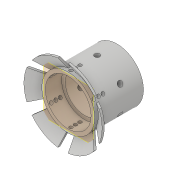
# Autodesk Inventor part: 01_Autofocus_Magnet_holder_v0
Saved by Autodesk Inventor 2019.4 (Build 234330000, 330)
## iProperties
Created: 2020-10-26
Part Number: 01_Autofocus_Magnet_holder_v0
Material: Generic
Document SubType Name: Modeling
Designer: diederichbenedict
Density: 1 g/cm^3
Appearance: Default
Author: diederichbenedict
Autodesk Inventor part; units mm, degrees
ref_plane "YZ Plane" through (0, 0, 0) normal (1, 0, 0) x (0, 1, 0)
ref_plane "XZ Plane" through (0, 0, 0) normal (0, 1, 0) x (-1, 0, 0)
ref_plane "XY Plane" through (0, 0, 0) normal (0, 0, 1) x (1, 0, 0)
ref_plane "Work Plane1" through (0, 0, 0) normal (0, 0, 1) x (1, 0, 0)
sketch "Sketch1" plane through (0, 0, 0) normal (0, 0, 1) x (1, 0, 0)
  circle A0 centre (0, 0) radius 12.5 construction
  circle A1 centre (0, 0) radius 12.65
  circle A2 centre (0, 0) radius 14.65
  point P0 (0, 0)
  dimension "d0" = 25.3
  dimension "d1" = 2
  constraints: 2 centre point, 1 coincident
  measures "d0" diameter of A1
  measures "d1" radial gap between concentric circles of A1 A2
ref_plane "Work Plane2" through (-12.5, -12.5, -9) normal (0, 0, -1) x (0, 1, 0)
extrude "Extrusion1" add sketch "Sketch1" against normal up to surface (9 mm away)
sketch "Sketch2" plane through (0, 0, -9) normal (0, 0, -1) x (-1, 0, 0)
  circle A0 centre (0, 0) radius 12.65 projected
  circle A1 centre (0, 0) radius 14.65 projected
  circle A2 centre (0, 0) radius 10.65
  point P0 (0, 0)
  dimension "d4" = 2
  constraints: 1 centre point
  measures "d4" radial gap between concentric circles of A0 A2
extrude "Extrusion2" add sketch "Sketch2" along normal blind 10 contours A0 | A1
sketch "Sketch3" plane through (0, 0, 0) normal (0, 1, 0) x (-1, 0, 0)
  line L0 (-9.95, -2) -> (9.95, -2) projected
  line L1 (-9.95, -4) -> (9.95, -4) projected
  line L2 (12.5, -6) -> (-12.5, -6) projected
  circle A0 centre (0, -1.5) radius 0.95
  line L3 (-12.65, 0) -> (12.65, 0) projected
  circle A1 centre (0, -4) radius 0.95
  circle A2 centre (0, -6.5) radius 0.95
  circle A3 centre (0, -16) radius 1.45
  line L4 (10.65, -19) -> (-10.65, -19) projected
  point P0 (0, 0)
  dimension "d7" = 1.9
  dimension "d8" = 1.5
  dimension "d9" = 1.9
  dimension "d10" = 2.5
  dimension "d11" = 1.9
  dimension "d12" = 2.5
  dimension "d31" = 2.9
  dimension "d32" = 3
  constraints: 4 centre point, 1 midpoint
  measures "d7" diameter of A0
  measures "d8" distance from line of A0.centre L3
  measures "d9" diameter of A1
  measures "d10" distance of A1.centre A0.centre
  measures "d11" diameter of A2
  measures "d12" distance of A2.centre A1.centre
  measures "d31" diameter of A3
  measures "d32" distance from line of A3.centre L4
extrude "Extrusion3" cut sketch "Sketch3" against normal through all
pattern_circular "Circular Pattern1" count 6 over 360 about axis through (0, 0, 0) along (0, 0, -1) of "Extrusion3"
sketch "Sketch4" plane through (0, 0, -19) normal (0, 0, -1) x (-1, 0, 0)
  circle A0 centre (0, 0) radius 10.65 construction
  circle A1 centre (0, 0) radius 14.65 construction
  line L0 (-9.5, -10.4) -> (-4, -10.4) construction
  line L1 (-9.5, -12.5) -> (-9.5, -10.4) construction
  line L2 (14.5, -12.5) -> (-9.5, -12.5) construction
  line L3 (14.5, 12.5) -> (14.5, -12.5) construction
  line L4 (-9.5, 12.5) -> (14.5, 12.5) construction
  line L5 (-9.5, 10.4) -> (-9.5, 12.5) construction
  line L6 (-4, 10.4) -> (-9.5, 10.4) construction
  line L7 (-4, -10.4) -> (-4, 10.4) construction
  circle A2 centre (12.5, -10.5) radius 1.05 construction
  circle A3 centre (0, -10.5) radius 1.05 construction
  circle A4 centre (0, 10.5) radius 1.05 construction
  circle A5 centre (12.5, 10.5) radius 1.05 construction
  line L8 (0.9, -9) -> (12.5, -9) construction
  line L9 (0.9, 8.7) -> (0.9, -9) construction
  line L10 (12.5, 8.7) -> (0.9, 8.7) construction
  line L11 (12.5, -9) -> (12.5, 8.7) construction
  line L12 (14.5, 2.0911) -> (14.5, -2.0911)
  circle A6 centre (0, 0) radius 14.65 projected
  arc A7 (7.6402, 12.5) -> (7.6402, -12.5) centre (0, 0) ccw
  circle A8 centre (0, 0) radius 10.65
  line L13 (-9.5, 11.1522) -> (-9.5, 12.5)
  line L14 (-9.5, -12.5) -> (-9.5, -11.1522)
  line L15 (14.5, -12.5) -> (7.6402, -12.5)
  line L16 (-7.6402, -12.5) -> (-9.5, -12.5)
  line L17 (-9.5, 12.5) -> (-7.6402, 12.5)
  line L18 (7.6402, 12.5) -> (14.5, 12.5)
  circle A9 centre (0, 0) radius 10.65 projected
  line L19 (5.6941, -9) -> (-5.6941, -9)
  line L20 (6.1427, 8.7) -> (-6.1427, 8.7)
  arc A10 (7.6402, -12.5) -> (14.5, -2.0911) centre (0, 0) ccw
  arc A11 (14.5, 2.0911) -> (7.6402, 12.5) centre (0, 0) ccw
  point P0 (0, 0)
  constraints: 22 point on circle, 20 end point, 7 parallel, 4 centre point, 4 perpendicular, 3 concentric, 3 point on line, 2 horizontal, 1 coincident
extrude "Extrusion4" add sketch "Sketch4" along normal blind 8 contours L12 A6 picked at (13.2167, 0)
sketch "Sketch5" plane through (0, 0, -27) normal (0, 0, -1) x (-1, 0, 0)
  circle A0 centre (12.5, -10.5) radius 1.05 projected
  circle A1 centre (12.5, 10.5) radius 1.05 projected
  circle A2 centre (0, 10.5) radius 1.05 projected
  circle A3 centre (0, -10.5) radius 1.05 projected
  point P0 (0, 0)
hole "Hole1" at (-12.5, -10.5, -27) at (-12.5, 10.5, -27) at (0, -10.5, -27) at (0, 10.5, -27) direction (0, 0, 1) diameter 1.5 depth 4 tip angle 118
sketch "Sketch6" plane through (0, 0, -27) normal (0, 0, -1) x (-1, 0, 0)
  line L0 (12.1017, 3.5) -> (8.4017, 3.5) projected
  line L1 (12.1017, -3.5) -> (8.4017, -3.5) projected
  circle A0 centre (0, 0) radius 6 projected
  line L2 (6.3468, 5.1817) -> (12.8864, 5.1817)
  line L3 (12.8864, 5.1817) -> (12.8864, -5.4004)
  line L4 (12.8864, -5.4004) -> (6.3468, -5.4004)
  line L5 (6.3468, -5.4004) -> (6.3468, 5.1817)
  line L6 (6.3468, 5.1817) -> (12.8864, -5.4004) construction
  line L7 (12.8864, 5.1817) -> (6.3468, -5.4004) construction
  point P0 (0, 0)
  point P1 (9.6166, -0.1093)
  constraints: 12 end point, 2 midpoint, 2 parallel, 1 horizontal, 1 perpendicular
extrude "Extrusion5" cut sketch "Sketch6" against normal blind 7 contours L2 L3 L4 L5
sketch "Sketch7" plane through (0, 0, -27) normal (0, 0, -1) x (-1, 0, 0)
  line L0 (9.3044, 5.1817) -> (12.8864, 5.1817) projected
  line L1 (12.8864, 5.1817) -> (12.8864, -5.4004) projected
  line L2 (12.8864, -5.4004) -> (9.1792, -5.4004) projected
  arc A0 (0.7396, -10.6243) -> (9.1792, -5.4004) centre (0, 0) ccw projected
  arc A1 (9.3044, 5.1817) -> (0.7396, 10.6243) centre (0, 0) ccw projected
  arc A2 (-0.7396, 10.6243) -> (-0.7396, -10.6243) centre (0, 0) ccw projected
  line L3 (14.5, -2.0911) -> (14.5, 2.0911) projected
  arc A3 (14.5, 2.0911) -> (14.5, -2.0911) centre (0, 0) ccw projected
  arc A4 (0.7396, 10.6243) -> (-0.7396, 10.6243) centre (0, 10.5) ccw projected
  arc A5 (-0.7396, -10.6243) -> (0.7396, -10.6243) centre (0, -10.5) ccw projected
  line L4 (5.7644, -8.9551) -> (7.6402, -12.5)
  line L5 (6.0377, -13.348) -> (3.7369, -9)
  line L6 (5.6941, -9) -> (-5.6941, -9) projected
  point P0 (0, 0)
  constraints: 4 end point, 2 point on circle, 1 parallel, 1 point on line
extrude "Extrusion6" cut sketch "Sketch7" against normal blind 7 contours L0 L1 L2 A0 L6 A2 A4 A1 | L6 L5 A0 A5 A2 | L6 A0 L5
sketch "Sketch8" plane through (0, 0, 0) normal (0, 1, 0) x (-1, 0, 0)
  line L0 (14.65, 0) -> (14.65, -19) projected
  line L1 (-14.65, 0) -> (-14.65, -27) projected
  line L2 (14.65, 0) -> (14.65, -19) projected
  line L3 (-14.65, 0) -> (14.65, 0) projected
  line L4 (-12.65, -9) -> (12.65, -9) projected
  line L5 (0, -32.9803) -> (0, 8.8817) projected
  line L6 (14.65, 0) -> (14.65, -19) projected
  line L7 (14.65, -2) -> (21.65, 2.9015)
  line L8 (14.65, -2) -> (23.1954, -2) construction
  line L9 (21.65, 2.9015) -> (21.65, 1.6807)
  line L10 (14.65, 0) -> (14.65, -19) projected
  line L11 (21.65, 1.6807) -> (14.65, -3.2208)
  line L12 (14.65, -3.2208) -> (14.65, -2)
  point P0 (0, 0)
  point P1 (17.6706, 0.115)
  point P2 (19.7184, 1.549)
  dimension "d41" = 35
  dimension "d43" = 1
  dimension "d44" = 2
  dimension "d45" = 7
  constraints: 10 end point, 3 point on line, 2 parallel, 1 equal length, 1 horizontal, 2 other
  measures "d41" angle of L8 L7
  measures "d43" distance between parallel lines of L11 L7
  measures "d44" distance of L7.start L2.start
  measures "d45" distance between parallel lines of L12 L9
revolve "Revolution1" add sketch "Sketch8" angle 45 mid plane about axis through (0, 0, -10) along (0, 0, 1)
pattern_circular "Circular Pattern2" count 6 over 360 about axis through (0, 0, 0) along (0, 0, -1) of "Revolution1"
sketch "Sketch9" plane through (0, 0, -27) normal (0, 0, -1) x (-1, 0, 0)
  arc A0 (0.7396, 10.6243) -> (-0.7396, 10.6243) centre (0, 10.5) ccw projected
  arc A1 (-0.7396, -10.6243) -> (0.7396, -10.6243) centre (0, -10.5) ccw projected
  circle A2 centre (0, 10.5) radius 0.75
  circle A3 centre (0, 0) radius 10.65 construction
  line L0 (-6.0081, 8.7935) -> (6.0081, 8.7935)
  line L1 (-6.0081, -8.7935) -> (6.0081, -8.7935)
  arc A4 (-0.7396, 10.6243) -> (-6.0081, 8.7935) centre (0, 0) ccw
  arc A5 (6.0081, 8.7935) -> (0.7396, 10.6243) centre (0, 0) ccw
  arc A6 (-6.0081, -8.7935) -> (-0.7396, -10.6243) centre (0, 0) ccw
  arc A7 (0.7396, -10.6243) -> (6.0081, -8.7935) centre (0, 0) ccw
  arc A8 (0.7396, -10.6243) -> (-0.7396, -10.6243) centre (0, -10.5) ccw
  point P0 (0, 0)
  dimension "d46" = 0
  constraints: 10 point on circle, 6 centre point, 4 end point, 2 concentric, 1 coincident, 1 horizontal, 1 parallel, 8 other
  measures "d46" horizontal distance of L1.start L0.start
extrude "Extrusion7" add sketch "Sketch9" against normal blind 3 contours A5 L0 A4 A2 | A6 L1 A7 A8
body "Solid1"
